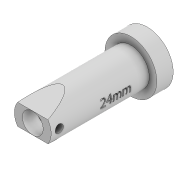
# Autodesk Inventor part: 200610 - 7-5mm lens adapter for half inch tube - sample side
Saved by Autodesk Inventor 2020.3 (Build 243373000, 373)
## iProperties
Created: 2020-06-10
Part Number: 200610 - 7-5mm lens adapter for half inch tube - sample side
Material: Generic
Document SubType Name: Modeling
Designer: Ralf
Density: 1 g/cm^3
Appearance: Default
Author: Ralf
Autodesk Inventor part; units mm, degrees
ref_plane "XZ Plane" through (0, 0, 0) normal (0, 1, 0) x (-1, 0, 0)
ref_plane "XY Plane" through (0, 0, 0) normal (0, 0, 1) x (1, 0, 0)
sketch "Sketch1" plane through (0, 0, 0) normal (0, 0, 1) x (1, 0, 0)
  circle A0 centre (0, 0) radius 6.35
  circle A1 centre (0, 0) radius 4
  dimension "d0" = 12.7
  dimension "d1" = 8
  constraints: 2 centre point, 2 coincident
  measures "d0" diameter of A0
  measures "d1" diameter of A1
extrude "Extrusion1" add sketch "Sketch1" along normal blind 4
sketch "Sketch2" plane through (0, 0, 4) normal (0, 0, 1) x (1, 0, 0)
  circle A0 centre (0, 0) radius 4.5
  dimension "d4" = 9
  constraints: 1 centre point, 1 coincident
  measures "d4" diameter of A0
extrude "Extrusion2" add sketch "Sketch2" along normal blind 24
sketch "Sketch3" plane through (0, 0, 28) normal (0, 0, 1) x (1, 0, 0)
  circle A0 centre (0, 0) radius 2.45
  dimension "d7" = 4.9
  constraints: 1 centre point, 1 coincident
  measures "d7" diameter of A0
extrude "Extrusion3" cut sketch "Sketch3" against normal blind 30
sketch "Sketch4" plane through (0, 0, 0) normal (1, 0, 0) x (0, 1, 0)
  line L0 (4.5, 28) -> (-4.5, 28) projected
  line L1 (0, 28) -> (2.55, 28)
  line L2 (2.55, 28) -> (4.5, 20.7225)
  line L3 (4.5, 4) -> (4.5, 28) projected
  line L4 (4.5, 20.7225) -> (4.5, 28)
  line L5 (2.55, 28) -> (4.5, 20.7225)
  line L6 (0, 28) -> (-2.55, 28)
  line L7 (-2.55, 28) -> (-4.5, 20.7225)
  line L8 (-4.5, 4) -> (-4.5, 28) projected
  line L9 (-4.5, 20.7225) -> (-4.5, 28)
  line L10 (-2.55, 28) -> (-4.5, 28)
  point P0 (0, 0)
  dimension "d10" = 2.55
  dimension "d11" = 105
  dimension "d14" = 2.55
  dimension "d15" = 105
  constraints: 16 end point, 6 point on line, 2 collinear, 1 midpoint, 1 perpendicular
  measures "d10" distance of L1.start L1.end
  measures "d11" angle of L1 L2
  measures "d14" distance of L1.start L6.end
  measures "d15" angle of L7 L6
extrude "Extrusion4" cut sketch "Sketch4" along normal mid plane 10
ref_plane "Work Plane1" through (4.5, 0, 0) normal (1, 0, 0) x (0, 1, 0)
sketch "Sketch6" plane through (4.5, 0, 0) normal (1, 0, 0) x (0, 1, 0)
  line L0 (1.104, 15.9988) -> (1.104, 10.9388) construction
  line L1 (1.104, 10.9388) -> (0.0618, 10.9388) construction
  line L2 (0.0618, 10.9388) -> (0.0618, 15.9988) construction
  line L3 (0.0618, 15.9988) -> (1.104, 15.9988) construction
  line L4 (-0.9382, 14.6196) -> (-0.9382, 15.8529)
  line L5 (-0.9382, 15.8529) -> (-0.6546, 15.8529)
  spline S0 degree 2 poles (-0.6546, 15.8529) (-0.5298, 15.72) (-0.298, 15.4834) (-0.1732, 15.37) knots 0 0 0 1 2 2 2
  spline S1 degree 2 poles (-0.1732, 15.37) (0.078, 15.1414) (0.3795, 14.9745) (0.5399, 14.9745) knots 0 0 0 1 2 2 2
  spline S2 degree 2 poles (0.5399, 14.9745) (0.6242, 14.9745) (0.7506, 15.0264) (0.7912, 15.0734) knots 0 0 0 1 2 2 2
  spline S3 degree 2 poles (0.7912, 15.0734) (0.8317, 15.1204) (0.8722, 15.2435) (0.8722, 15.3181) knots 0 0 0 1 2 2 2
  spline S4 degree 2 poles (0.8722, 15.3181) (0.8722, 15.3894) (0.8365, 15.5353) (0.809, 15.6017) knots 0 0 0 1 2 2 2
  spline S5 degree 2 poles (0.809, 15.6017) (0.7863, 15.6584) (0.7215, 15.7638) (0.6988, 15.7962) knots 0 0 0 1 2 2 2
  line L6 (0.6988, 15.7962) -> (0.6988, 15.8108)
  line L7 (0.6988, 15.8108) -> (0.984, 15.8108)
  spline S6 degree 2 poles (0.984, 15.8108) (1.0245, 15.7281) (1.104, 15.4315) (1.104, 15.2986) knots 0 0 0 1 2 2 2
  spline S7 degree 2 poles (1.104, 15.2986) (1.104, 15.0183) (0.8074, 14.7022) (0.5545, 14.7022) knots 0 0 0 1 2 2 2
  spline S8 degree 2 poles (0.5545, 14.7022) (0.4362, 14.7022) (0.2385, 14.7573) (0.1542, 14.8059) knots 0 0 0 1 2 2 2
  spline S9 degree 2 poles (0.1542, 14.8059) (0.0667, 14.8546) (-0.1051, 14.9956) (-0.1878, 15.0734) knots 0 0 0 1 2 2 2
  spline S10 degree 2 poles (-0.1878, 15.0734) (-0.3255, 15.1998) (-0.6205, 15.5093) (-0.7064, 15.6017) knots 0 0 0 1 2 2 2
  line L8 (-0.7064, 15.6017) -> (-0.7064, 14.6196)
  line L9 (-0.7064, 14.6196) -> (-0.9382, 14.6196)
  line L10 (-0.251, 13.0653) -> (-0.251, 13.3035)
  line L11 (-0.251, 13.3035) -> (-0.9382, 13.3035)
  line L12 (-0.9382, 13.3035) -> (-0.9382, 13.5612)
  line L13 (-0.9382, 13.5612) -> (-0.251, 13.5612)
  line L14 (-0.251, 13.5612) -> (-0.251, 14.4445)
  line L15 (-0.251, 14.4445) -> (0.031, 14.4445)
  line L16 (0.031, 14.4445) -> (1.0618, 13.5499)
  line L17 (1.0618, 13.5499) -> (1.0618, 13.3035)
  line L18 (1.0618, 13.3035) -> (-0.0354, 13.3035)
  line L19 (-0.0354, 13.3035) -> (-0.0354, 13.0653)
  line L20 (-0.0354, 13.0653) -> (-0.251, 13.0653)
  line L21 (-0.0354, 13.5612) -> (0.7458, 13.5612)
  line L22 (0.7458, 13.5612) -> (-0.0354, 14.2338)
  line L23 (-0.0354, 14.2338) -> (-0.0354, 13.5612)
  line L24 (-0.9382, 11.1123) -> (-0.0695, 11.1123)
  spline S11 degree 2 poles (-0.0695, 11.1123) (0.0343, 11.1123) (0.2109, 11.1285) (0.2595, 11.1544) knots 0 0 0 1 2 2 2
  spline S12 degree 2 poles (0.2595, 11.1544) (0.313, 11.1803) (0.3649, 11.2792) (0.3649, 11.3651) knots 0 0 0 1 2 2 2
  spline S13 degree 2 poles (0.3649, 11.3651) (0.3649, 11.4429) (0.2693, 11.6212) (0.1785, 11.7152) knots 0 0 0 1 2 2 2
  spline S14 degree 2 poles (0.1785, 11.7152) (0.1558, 11.7136) (0.0926, 11.7103) (0.0505, 11.7103) knots 0 0 0 1 2 2 2
  line L25 (0.0505, 11.7103) -> (-0.9382, 11.7103)
  line L26 (-0.9382, 11.7103) -> (-0.9382, 11.9631)
  line L27 (-0.9382, 11.9631) -> (-0.0695, 11.9631)
  spline S15 degree 2 poles (-0.0695, 11.9631) (0.0343, 11.9631) (0.2109, 11.9794) (0.2595, 12.0053) knots 0 0 0 1 2 2 2
  spline S16 degree 2 poles (0.2595, 12.0053) (0.313, 12.0312) (0.3649, 12.1301) (0.3649, 12.216) knots 0 0 0 1 2 2 2
  spline S17 degree 2 poles (0.3649, 12.216) (0.3649, 12.297) (0.2628, 12.4769) (0.1834, 12.5612) knots 0 0 0 1 2 2 2
  line L28 (0.1834, 12.5612) -> (-0.9382, 12.5612)
  line L29 (-0.9382, 12.5612) -> (-0.9382, 12.814)
  line L30 (-0.9382, 12.814) -> (0.5626, 12.814)
  line L31 (0.5626, 12.814) -> (0.5626, 12.5612)
  line L32 (0.5626, 12.5612) -> (0.3973, 12.5612)
  spline S18 degree 2 poles (0.3973, 12.5612) (0.4962, 12.4623) (0.6048, 12.2679) (0.6048, 12.1512) knots 0 0 0 1 2 2 2
  spline S19 degree 2 poles (0.6048, 12.1512) (0.6048, 12.0183) (0.4832, 11.8124) (0.3454, 11.7589) knots 0 0 0 1 2 2 2
  spline S20 degree 2 poles (0.3454, 11.7589) (0.4735, 11.6439) (0.6048, 11.4267) (0.6048, 11.3003) knots 0 0 0 1 2 2 2
  spline S21 degree 2 poles (0.6048, 11.3003) (0.6048, 11.203) (0.5448, 11.0442) (0.4767, 10.9858) knots 0 0 0 1 2 2 2
  spline S22 degree 2 poles (0.4767, 10.9858) (0.4087, 10.9259) (0.2044, 10.8594) (0.0505, 10.8594) knots 0 0 0 1 2 2 2
  line L33 (0.0505, 10.8594) -> (-0.9382, 10.8594)
  line L34 (-0.9382, 10.8594) -> (-0.9382, 11.1123)
  line L35 (-0.9382, 8.8027) -> (-0.0695, 8.8027)
  spline S23 degree 2 poles (-0.0695, 8.8027) (0.0343, 8.8027) (0.2109, 8.8189) (0.2595, 8.8448) knots 0 0 0 1 2 2 2
  spline S24 degree 2 poles (0.2595, 8.8448) (0.313, 8.8708) (0.3649, 8.9696) (0.3649, 9.0555) knots 0 0 0 1 2 2 2
  spline S25 degree 2 poles (0.3649, 9.0555) (0.3649, 9.1333) (0.2693, 9.3116) (0.1785, 9.4056) knots 0 0 0 1 2 2 2
  spline S26 degree 2 poles (0.1785, 9.4056) (0.1558, 9.404) (0.0926, 9.4008) (0.0505, 9.4008) knots 0 0 0 1 2 2 2
  line L36 (0.0505, 9.4008) -> (-0.9382, 9.4008)
  line L37 (-0.9382, 9.4008) -> (-0.9382, 9.6536)
  line L38 (-0.9382, 9.6536) -> (-0.0695, 9.6536)
  spline S27 degree 2 poles (-0.0695, 9.6536) (0.0343, 9.6536) (0.2109, 9.6698) (0.2595, 9.6957) knots 0 0 0 1 2 2 2
  spline S28 degree 2 poles (0.2595, 9.6957) (0.313, 9.7217) (0.3649, 9.8205) (0.3649, 9.9064) knots 0 0 0 1 2 2 2
  spline S29 degree 2 poles (0.3649, 9.9064) (0.3649, 9.9875) (0.2628, 10.1674) (0.1834, 10.2516) knots 0 0 0 1 2 2 2
  line L39 (0.1834, 10.2516) -> (-0.9382, 10.2516)
  line L40 (-0.9382, 10.2516) -> (-0.9382, 10.5045)
  line L41 (-0.9382, 10.5045) -> (0.5626, 10.5045)
  line L42 (0.5626, 10.5045) -> (0.5626, 10.2516)
  line L43 (0.5626, 10.2516) -> (0.3973, 10.2516)
  spline S30 degree 2 poles (0.3973, 10.2516) (0.4962, 10.1528) (0.6048, 9.9583) (0.6048, 9.8416) knots 0 0 0 1 2 2 2
  spline S31 degree 2 poles (0.6048, 9.8416) (0.6048, 9.7087) (0.4832, 9.5029) (0.3454, 9.4494) knots 0 0 0 1 2 2 2
  spline S32 degree 2 poles (0.3454, 9.4494) (0.4735, 9.3343) (0.6048, 9.1171) (0.6048, 8.9907) knots 0 0 0 1 2 2 2
  spline S33 degree 2 poles (0.6048, 8.9907) (0.6048, 8.8935) (0.5448, 8.7346) (0.4767, 8.6763) knots 0 0 0 1 2 2 2
  spline S34 degree 2 poles (0.4767, 8.6763) (0.4087, 8.6163) (0.2044, 8.5499) (0.0505, 8.5499) knots 0 0 0 1 2 2 2
  line L44 (0.0505, 8.5499) -> (-0.9382, 8.5499)
  line L45 (-0.9382, 8.5499) -> (-0.9382, 8.8027)
  point P0 (0, 0)
  constraints: 2 other
extrude "Extrusion5" cut sketch "Sketch6" against normal blind 0.5
sketch "Sketch8" plane through (0, 0, 28) normal (0, 0, 1) x (1, 0, 0)
  circle A0 centre (0, 0) radius 2.55
  dimension "d21" = 5.1
  constraints: 1 centre point, 1 coincident
  measures "d21" diameter of A0
extrude "Extrusion6" cut sketch "Sketch8" against normal blind 3.5
sketch "Sketch7" plane through (4.5, 0, 0) normal (1, 0, 0) x (0, 1, 0)
  circle A0 centre (0, 26) radius 1
  line L0 (2.55, 28) -> (-2.55, 28) projected
  point P0 (0, 0)
  dimension "d19" = 2
  dimension "d20" = 2
  constraints: 1 centre point
  measures "d19" diameter of A0
  measures "d20" distance from line of A0.centre L0
extrude "Extrusion7" cut sketch "Sketch7" against normal blind 5
body "Solid1"
